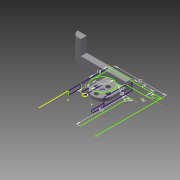
# Autodesk Inventor part: CraneGripper
Saved by Autodesk Inventor 2015 (Build 190159000, 159)
## iProperties
Created: 2016-03-24
Part Number: CraneGripper
Material: Generic
Document SubType Name: Modeling
Designer: Hatch
Density: 1 g/cm^3
Appearance: Default
Author: Hatch
Autodesk Inventor part; units mm, degrees
ref_plane "YZ Plane" through (0, 0, 0) normal (1, 0, 0) x (0, 1, 0)
ref_plane "XZ Plane" through (0, 0, 0) normal (0, 1, 0) x (-1, 0, 0)
ref_plane "XY Plane" through (0, 0, 0) normal (0, 0, 1) x (1, 0, 0)
sketch "Sketch1" plane through (0, 0, 0) normal (0, 1, 0) x (-1, 0, 0)
  line L0 (0, 0) -> (24, 0)
  line L1 (12, 0) -> (12, -5)
  circle A0 centre (12, -5) radius 2.125
  dimension "d0" = 24
  dimension "d1" = 5
  dimension "d2" = 4.25
  constraints: 4 end point, 1 centre point, 1 coincident, 1 horizontal, 1 midpoint, 1 vertical
  measures "d0" distance of L0.start L0.end
  measures "d1" distance of L1.start L1.end
  measures "d2" diameter of A0
sketch "Sketch2" plane through (0, 0, 0) normal (0, 1, 0) x (-1, 0, 0)
  line L0 (24, 0) -> (24, 30)
  line L1 (24, 30) -> (0, 30)
  line L2 (0, 0) -> (0, -12.5)
  line L3 (0, -12.5) -> (24, -12.5)
  line L4 (24, -12.5) -> (24, 0)
  line L5 (0, 25) -> (0, 0)
  line L6 (0, 25) -> (-29.86, 25)
  line L7 (0, 30) -> (-29.86, 30)
  line L8 (-29.86, 30) -> (-29.86, 25)
  dimension "d3" = 24
  dimension "d4" = 30
  dimension "d5" = 12.5
  dimension "d6" = 5
  dimension "d20" = 29.86
  constraints: 18 end point, 3 horizontal, 2 perpendicular, 1 collinear
  measures "d3" distance of L2.start L0.start
  measures "d4" distance of L0.start L0.end
  measures "d5" distance of L2.start L2.end
  measures "d6" distance of L1.end L5.start
  measures "d20" distance of L5.start L6.end
extrude "Extrusion1" add sketch "Sketch2" along normal blind 8
extrude "Extrusion2" cut sketch "Sketch1" along normal through all
pattern_linear "Rectangular Pattern1" count 2 spacing 6 along (1, 0, 0) count 2 spacing 6 along (-1, 0, 0) of "Extrusion2"
sketch "Sketch4" plane through (-24, 0, -12.5) normal (-1, 0, 0) x (0, 0, 1)
  point P0 (12.5, 0)
sketch "Sketch5" plane through (0, 8, 0) normal (0, 1, 0) x (1, 0, 0)
  line L0 (0, 0) -> (0, 12.5)
  line L1 (0, 12.5) -> (-24, 12.5)
  line L2 (-24, 12.5) -> (-24, 0)
  line L3 (-24, 0) -> (0, 0)
  line L4 (0, -25) -> (0, 12.5) projected
  constraints: 8 end point, 2 parallel, 1 collinear, 1 perpendicular
extrude "Extrusion3" cut sketch "Sketch5" against normal blind 5
sketch "Sketch6" plane through (0, 8, 0) normal (0, 1, 0) x (1, 0, 0)
  line L0 (13.1425, -25) -> (13.1425, 25)
  circle A0 centre (-12, 5) radius 2.125 projected
  line L1 (-12, 5) -> (-12, 23)
  circle A1 centre (-12, 23) radius 10
  line L2 (21.1928, 30) -> (23.1928, 30)
  line L3 (0, 35) -> (20, 35)
  line L4 (20, 35) -> (30.8046, 35) construction
  line L5 (20, 35) -> (37.0437, 35) construction
  line L6 (20, 35) -> (24.8301, 36.2923)
  line L7 (17.3205, 25) -> (22.3205, 25) construction
  line L8 (17.3205, 25) -> (12.3205, 25)
  line L9 (-2, 23) -> (0, 35)
  line L10 (-22, 23) -> (-22, 41)
  line L11 (-22, 41) -> (30, 41)
  line L12 (30, 41) -> (24.8301, 36.2923)
  point P0 (0, 0)
  dimension "d23" = 50
  dimension "d25" = 18
  dimension "d26" = 20
  dimension "d42" = 2
  dimension "d45" = 20
  dimension "d47" = 20
  dimension "d52" = 5
  dimension "d63" = 5
  dimension "d66" = 52
  dimension "d67" = 18
  constraints: 26 end point, 3 horizontal, 3 vertical, 2 point on circle, 1 centre point, 1 perpendicular
  measures "d23" distance of L0.start L0.end
  measures "d25" distance of L1.start L1.end
  measures "d26" diameter of A1
  measures "d42" distance of L2.start L2.end
  measures "d45" distance of L3.start L3.end
  measures "d47" distance of L3.start L7.start
  measures "d52" distance of L3.end L6.end
  measures "d63" distance of L7.start L8.end
  measures "d66" distance of L10.end L11.end
  measures "d67" distance of L10.start L10.end
sketch "Sketch7" plane through (0, 0, 0) normal (0, -1, 0) x (1, 0, 0)
  circle A0 centre (-12, -5) radius 2.125 projected
  line L0 (-12, -5) -> (-12, -23)
  circle A1 centre (-12, -23) radius 10
  line L1 (-22, -23) -> (-22, -41)
  line L2 (-22, -41) -> (30, -41)
  line L3 (0, -34.9999) -> (20, -34.9999)
  line L4 (20, -34.9999) -> (24.851, -36.2115)
  line L5 (24.851, -36.2115) -> (30, -41)
  line L6 (0, -34.9999) -> (-2, -23)
  point P0 (0, 0)
  dimension "d27" = 18
  dimension "d28" = 20
  dimension "d68" = 18
  dimension "d69" = 52
  dimension "d70" = 20
  dimension "d71" = 5
  constraints: 14 end point, 2 point on circle, 2 vertical, 1 centre point, 1 coincident, 1 horizontal, 1 perpendicular, 1 tangent
  measures "d27" distance of L0.start L0.end
  measures "d28" diameter of A1
  measures "d68" distance of L1.start L1.end
  measures "d69" distance of L1.end L2.end
  measures "d70" distance of L3.start L3.end
  measures "d71" distance of L3.end L4.end
extrude "Extrusion4" add sketch "Sketch7" against normal blind 3 contours A1
sketch "Sketch8" plane through (-12, 3, -23) normal (0, 1, 0) x (1, 0, 0)
  circle A0 centre (0, 0) radius 2.125
  point P0 (12, -23)
  dimension "d31" = 4.25
  constraints: 1 centre point
  measures "d31" diameter of A0
extrude "Extrusion5" cut sketch "Sketch8" against normal blind 1
sketch "Sketch9" plane through (-12, 3, -23) normal (0, 1, 0) x (1, 0, 0)
  line L0 (0, 0) -> (-6, 0)
  circle A0 centre (-6, 0) radius 2.125
  point P0 (12, -23)
  dimension "d34" = 6
  dimension "d35" = 4.25
  constraints: 2 end point, 1 centre point, 1 coincident, 1 horizontal
  measures "d34" distance of L0.start L0.end
  measures "d35" diameter of A0
extrude "Extrusion6" cut sketch "Sketch9" against normal through all
pattern_circular "Circular Pattern1" count 4 over 360 about axis through (-12, 0, -23) along (0, 1, 0) of "Extrusion6"
sketch "Sketch10" plane through (-12, 0, -23) normal (0, -1, 0) x (1, 0, 0)
  circle A0 centre (0, 0) radius 10 projected
  line L0 (-10, 0) -> (-10, -18)
  line L1 (-10, -18) -> (42, -18)
  line L2 (12, -12) -> (32, -12)
  line L3 (32, -12) -> (36.8295, -13.2918)
  line L4 (36.8295, -13.2918) -> (42, -18)
  arc A1 (-10, 0) -> (10, 0) centre (0, 0) ccw
  line L5 (10, 0) -> (12, -12)
  point P0 (12, 23)
  dimension "d72" = 18
  dimension "d73" = 52
  dimension "d74" = 20
  constraints: 12 end point, 2 point on circle, 2 vertical, 1 centre point, 1 coincident, 1 horizontal, 1 horizontal alignment, 1 perpendicular, 2 other
  measures "d72" distance of L0.start L0.end
  measures "d73" distance of L0.end L1.end
  measures "d74" distance of L2.start L2.end
extrude "Extrusion7" add sketch "Sketch10" against normal blind 8 contours L5 L2 L3 L4 L1 L0 A0
sketch "Sketch11" plane through (0, 0, 25) normal (1, 0, 0) x (0, 0, -1)
  line L0 (25, 8) -> (37.5, 8)
  line L1 (37.5, 8) -> (37.5, 4)
  line L2 (37.5, 4) -> (25, 4)
  line L3 (25, 4) -> (25, 8)
  point P0 (25, 0)
  dimension "d77" = 4
  constraints: 8 end point, 2 parallel, 1 horizontal, 1 perpendicular
  measures "d77" distance of L0.end L1.end
extrude "Extrusion8" add sketch "Sketch11" against normal blind 24
sketch "Sketch12" plane through (0, 8, 0) normal (0, 1, 0) x (1, 0, 0)
  circle A0 centre (-12, 5) radius 2.125 projected
  circle A1 centre (-12, 5) radius 2.125
  point P0 (0, 0)
  dimension "d80" = 4.25
  constraints: 1 centre point, 1 coincident
  measures "d80" diameter of A1
extrude "Extrusion9" cut sketch "Sketch12" against normal through all
pattern_linear "Rectangular Pattern2" count 3 spacing 6 along (1, 0, 0) of "Extrusion9"
sketch "Sketch13" plane through (0, 8, 0) normal (0, 1, 0) x (1, 0, 0)
  line L0 (30, 41) -> (29.8598, -25)
  point P0 (0, 0)
  point P1 (29.86, -25)
  constraints: 2 end point
fillet "Fillet1" radius 5 1 edges at (29.86, 4, 30)
sketch "Sketch14" plane through (0, 0, 25) normal (1, 0, 0) x (0, 0, -1)
  line L0 (37.5, 3) -> (25, 3)
  line L1 (25, 3) -> (25, 0)
  line L2 (25, 0) -> (37.5, 0)
  line L3 (37.5, 0) -> (37.5, 3)
  line L4 (37.5, 0) -> (66, 0)
  line L5 (66, 0) -> (66, 8)
  line L6 (66, 8) -> (37.5, 8)
  line L7 (37.5, 8) -> (37.5, 0)
  constraints: 16 end point, 4 parallel, 2 horizontal, 2 perpendicular
sketch "Sketch15" plane through (0, 0, 25) normal (1, 0, 0) x (0, 0, -1)
  point P0 (25, 0)
sketch "Sketch16" plane through (-24, 0, -12.5) normal (-1, 0, 0) x (0, 0, 1)
  line L0 (0, 8) -> (42.5, 8) projected
  line L1 (0, 4) -> (12.5, 4)
  line L2 (12.5, 4) -> (12.5, 8)
  line L3 (12.5, 8) -> (0, 8)
  line L4 (0, 8) -> (0, 4)
  line L5 (-0.5, 0) -> (-10.5, 0) projected
  line L6 (-0.5431, 0) -> (-28.5, 0)
  line L7 (-28.5, 0) -> (-28.5, 8)
  line L8 (-28.5, 8) -> (-0.5431, 8)
  line L9 (-0.5431, 8) -> (-0.5431, 0)
  point P0 (12.5, 0)
  constraints: 16 end point, 4 parallel, 2 horizontal, 2 perpendicular, 2 point on line
sketch "Sketch17" plane through (0, 8, 0) normal (0, 1, 0) x (1, 0, 0)
  line L0 (-28.6904, -36.0385) -> (31.2177, -36.0385)
  line L1 (31.2177, -36.0385) -> (31.2177, 12.5)
  line L2 (31.2177, 12.5) -> (-28.6904, 12.5)
  line L3 (-28.6904, 12.5) -> (-28.6904, -36.0385)
  point P0 (0, 0)
  constraints: 8 end point, 2 parallel, 1 horizontal, 1 perpendicular
extrude "Extrusion10" cut sketch "Sketch17" against normal through all
sketch "Sketch18" plane through (-12, 8, -23) normal (0, 1, 0) x (1, 0, 0)
  line L0 (12, 12) -> (12, 14)
  line L1 (12, 14) -> (-10, 14)
  line L2 (-10, 14) -> (-10, 0)
  line L3 (-10, 0) -> (12, 0)
  line L4 (12, 0) -> (12, 14)
  point P0 (12, -23)
  dimension "d89" = 2
  constraints: 10 end point, 2 parallel, 1 horizontal, 1 perpendicular, 1 vertical
  measures "d89" distance of L0.start L0.end
extrude "Extrusion11" cut sketch "Sketch18" against normal blind 5
sketch "Sketch19" plane through (-22, 0, -41) normal (-1, 0, 0) x (0, 0, 1)
  line L0 (0, 0) -> (-2, 0)
  line L1 (-2, 0) -> (-2, 8)
  line L2 (-2, 8) -> (0, 8)
  line L3 (0, 8) -> (0, 0)
  point P0 (41, 0)
  dimension "d92" = 2
  constraints: 8 end point, 2 parallel, 1 horizontal, 1 perpendicular
  measures "d92" distance of L1.end L2.end
extrude "Extrusion12" add sketch "Sketch19" against normal blind 20
sketch "Sketch20" plane through (-12, 8, -23) normal (0, 1, 0) x (1, 0, 0)
  line L0 (10, 20) -> (42.0506, 20)
  line L1 (42.0506, 20) -> (42.0506, 0.0873)
  line L2 (42.0506, 0.0873) -> (10, 0.0873)
  line L3 (10, 0.0873) -> (10, 20)
  point P0 (12, -23)
  constraints: 8 end point, 2 parallel, 1 horizontal, 1 perpendicular
extrude "Extrusion13" cut sketch "Sketch20" against normal through all
sketch "Sketch21" plane through (-22, 0, -23) normal (-1, 0, 0) x (0, 0, 1)
  line L0 (-20, 0) -> (-14, 0)
  line L1 (-14, 0) -> (-14, 8)
  line L2 (-14, 8) -> (-20, 8)
  line L3 (-20, 8) -> (-20, 0)
  point P0 (23, 0)
  constraints: 8 end point, 2 parallel, 1 horizontal, 1 perpendicular
extrude "Extrusion14" add sketch "Sketch21" along normal blind 35
sketch "Sketch22" plane through (0, 0, 0) normal (0, -1, 0) x (1, 0, 0)
  point P0 (0, 0)
fillet "Fillet2" radius 6 1 edges at (-57, 4, -37)
sketch "Sketch24" plane through (-12, 8, -23) normal (0, 1, 0) x (1, 0, 0)
  arc A0 (-45, 20) -> (-39, 14) centre (-39, 20) ccw
  line L0 (-39, 14) -> (-36, 14)
  line L1 (-10, 14) -> (-39, 14) projected
  line L2 (-36, 14) -> (-36, 20)
  line L3 (-45, 20) -> (10, 20) projected
  point P0 (12, -23)
  dimension "d101" = 3
  constraints: 4 end point, 2 point on circle, 2 point on line, 1 centre point, 1 perpendicular
  measures "d101" distance of L0.start L0.end
extrude "Extrusion15" add sketch "Sketch24" along normal blind 15
equation "\"d81\" = d80"
body "Solid1"
